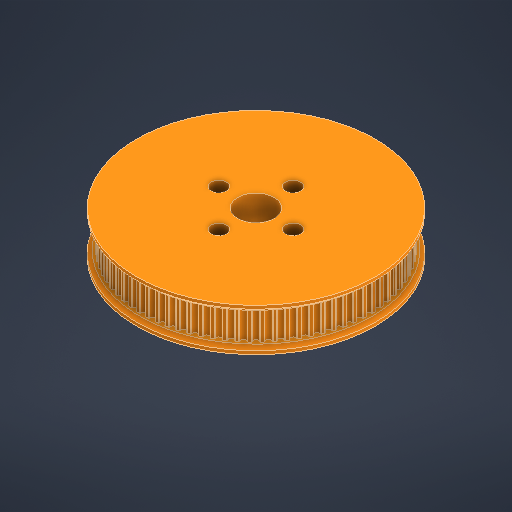
# Autodesk Inventor part: Engranaje insertado en PIN
Saved by Autodesk Inventor 2026 (Build 300175050, 175E)
## iProperties
Created: 2025-07-19
Part Number: Engranaje insertado en PIN
Material: Plastico PETG
Document SubType Name: Modeling
Designer: bello
Density: 1.27 g/cm^3
Appearance: Naranja
Author: bello
Autodesk Inventor part; units mm, degrees
ref_plane "YZ Plane" through (0, 0, 0) normal (1, 0, 0) x (0, 1, 0)
ref_plane "XZ Plane" through (0, 0, 0) normal (0, 1, 0) x (-1, 0, 0)
ref_plane "XY Plane" through (0, 0, 0) normal (0, 0, 1) x (1, 0, 0)
sketch "Boceto1" plane through (0, 0, 0) normal (0, 1, 0) x (-1, 0, 0)
  circle A0 centre (0, 0) radius 25.2108
  circle A1 centre (0, 0) radius 24.4608
  line L0 (0, 0) -> (0, -25.2108)
  line L1 (0, 0) -> (-1.978, -25.1331)
  circle A2 centre (0, -25.0158) radius 0.555
  circle A3 centre (-1.9627, -24.9387) radius 0.555
  circle A4 centre (-0.7041, -25.0509) radius 0.15
  circle A5 centre (-1.2635, -25.0289) radius 0.15
  circle A6 centre (0, 0) radius 22.4608
  point P0 (0, -22.4608)
  point P1 (-1.7623, -22.3916)
  point P2 (-1.9192, -24.3854)
  point P3 (-1.4123, -25.0097)
  point P4 (-1.2711, -25.1787)
  point P5 (-0.7083, -25.2008)
  point P6 (-0.5543, -25.0434)
  point P7 (0, -24.4608)
  dimension "d0" = 50.4216
  dimension "d1" = 48.9216
  dimension "d2" = 4.5
  dimension "d3" = 1.11
  dimension "d4" = 0.3
  dimension "d5" = 44.9216
  constraints: 7 centre point, 6 tangent, 4 end point, 3 coincident, 2 equal radius, 2 point on circle, 2 point on line, 1 vertical
  measures "d0" diameter of A0
  measures "d1" diameter of A1
  measures "d2" angle of L0 L1
  measures "d3" diameter of A2
  measures "d4" diameter of A4
  measures "d5" diameter of A6
extrude "Extrusión1" add sketch "Boceto1" along normal blind 6.5 contours L1 A6 L0 A1 | A1 A2 A4 A0 A5 A3 | L1 L0 A6 | A5 picked at (-1.6539, -23.7347) picked at (-0.196, -14.9713)
pattern_circular "Patrón circular1" count 80 over 360 about axis through (0, -10, 0) along (0, 1, 0) of "Extrusión1"
sketch "Boceto2" plane through (0, 6.5, 0) normal (0, 1, 0) x (1, 0, 0)
  circle A0 centre (0, 0) radius 26.5
  dimension "d11" = 53
  constraints: 1 centre point, 1 coincident
  measures "d11" diameter of A0
extrude "Extrusión2" add sketch "Boceto2" along normal blind 1.5
sketch "Boceto3" plane through (0, 0, 0) normal (0, -1, 0) x (1, 0, 0)
  circle A0 centre (0, 0) radius 26.5
  constraints: 1 centre point, 1 coincident
extrude "Extrusión3" add sketch "Boceto3" along normal blind 1.5
sketch "Boceto4" plane through (0, -1.5, 0) normal (0, -1, 0) x (1, 0, 0)
  circle A0 centre (0, 0) radius 12.55
  dimension "d16" = 25.1
  constraints: 1 centre point, 1 coincident
  measures "d16" diameter of A0
extrude "Extrusión4" add sketch "Boceto4" along normal blind 9
sketch "Boceto5" plane through (0, -1.5, 0) normal (0, -1, 0) x (1, 0, 0)
  circle A0 centre (0, 0) radius 14.5
  dimension "d19" = 29
  constraints: 1 centre point, 1 coincident
  measures "d19" diameter of A0
extrude "Extrusión5" add sketch "Boceto5" along normal blind 2
sketch "Boceto6" plane through (0, -10.5, 0) normal (0, -1, 0) x (1, 0, 0)
  circle A0 centre (0, 0) radius 4.05
  dimension "d22" = 8.1
  constraints: 1 centre point, 1 coincident
  measures "d22" diameter of A0
extrude "Extrusión6" cut sketch "Boceto6" against normal through all
chamfer "Chaflán1" distance 0.75 angle 45 2 edges at (-26.5, 0, 0) (-26.5, 6.5, 0)
sketch "Boceto8" plane through (0, -10.5, 0) normal (0, -1, 0) x (1, 0, 0)
  circle A0 centre (0, 0) radius 8.25
  circle A1 centre (8.25, 0) radius 1.7
  circle A2 centre (0, -8.25) radius 1.7
  circle A3 centre (-8.25, 0) radius 1.7
  circle A4 centre (0, 8.25) radius 1.7
  dimension "d28" = 3.4
  dimension "d29" = 16.5
  constraints: 5 centre point, 4 point on circle, 3 equal radius, 1 coincident
  measures "d28" diameter of A2
  measures "d29" diameter of A0
extrude "Extrusión7" cut sketch "Boceto8" against normal through all contours A0 A1 | A0 A1 | A4 A0 | A0 A4 | A2 A0 | A0 A2 | A3 A0 | A0 A3
equation "\"d0\" = PitchDiameter"
equation "\"d1\" = InnerDiameter"
equation "\"d2\" = ToothAngle"
equation "\"d3\" = RootDiameter"
equation "\"d4\" = ShoulderDiameter"
equation "\"Pitch\" = 2"
equation "\"InnerDiameter\" = PitchDiameter - 2 * ToothHeight"
equation "\"PitchDiameter\" = PulleyDiameter - 2 * PLD"
equation "\"PLD\" = 0.254"
equation "\"ToothHeight\" = 0.75"
equation "\"ShoulderDiameter\" = 0.3"
equation "\"RootDiameter\" = 1.11"
equation "\"ToothAngle\" = 4.5deg"
equation "\"PulleyDiameter\" = 50.929582"
